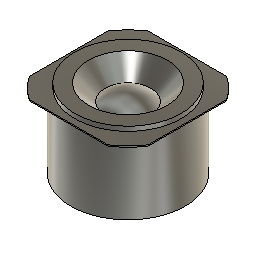
bc-4ndf34_phase_mount - thicker v5 v2 (Autodesk Fusion 360 archive; units mm, degrees)
design "bc-4ndf34-outline-parameterised"
Autodesk Fusion 360 part; units mm, degrees
sketch "Front frame" plane through (0, 0, 0) normal (0, 0, 1) x (1, 0, 0)
  line L0 (34.975, -53) -> (-34.975, -53)
  line L1 (-53, -34.975) -> (-53, 34.975)
  line L2 (-34.975, 53) -> (34.975, 53)
  line L3 (53, 34.975) -> (53, -34.975)
  line L4 (53, -53) -> (-53, 53) construction
  line L5 (-53, -53) -> (53, 53) construction
  arc A0 (53, 34.975) -> (34.975, 53) centre (0, 0) ccw
  arc A1 (53, 22.2991) -> (22.2991, 53) centre (0, 0) ccw
  arc A2 (34.975, -53) -> (53, -34.975) centre (0, 0) ccw
  arc A3 (22.2991, -53) -> (53, -22.2991) centre (0, 0) ccw
  arc A4 (-34.975, 53) -> (-53, 34.975) centre (0, 0) ccw
  arc A5 (-53, -34.975) -> (-34.975, -53) centre (0, 0) ccw
  arc A6 (-22.2991, 53) -> (-53, 22.2991) centre (0, 0) ccw
  arc A7 (-53, -22.2991) -> (-22.2991, -53) centre (0, 0) ccw
  circle A8 centre (0, 0) radius 51
  dimension "d1" = 127
  dimension "d2" = 115
  dimension "d3" = 106
  dimension "d4" = 106
  dimension "d15" = 102
  constraint coincident A0.centre A1.centre
  constraint horizontal L0
  constraint perpendicular L0 L1
  constraint parallel L0 L2
  constraint parallel L1 L3
  constraint coincident L4 A0.centre
  constraint coincident L5 A0.centre
  constraint coincident L2 A1.end
  constraint coincident L2 A6.start
  constraint coincident L3.start A4
  constraint concentric A0 A4
  constraint coincident L3 A3.end
  constraint coincident L3 A1.start
  constraint concentric A1 A6
  constraint coincident L0.start A4
  constraint concentric A2 A4
  constraint coincident L0 A7.end
  constraint coincident L0 A3.start
  constraint concentric A3 A6
  constraint coincident L1.start A4
  constraint concentric A4 A5
  constraint coincident L1 A6.end
  constraint coincident L1 A7.start
  constraint concentric A6 A7
  constraint concentric A4 A8
  measures "d1" diameter of A4
  measures "d2" diameter of A6
  measures "d3" distance of L4.end L5.end
  measures "d4" distance of L5.start L4.end
  measures "d15" diameter of A8
sketch "Side frame" plane through (0, 0, 0) normal (0, 1, 0) x (1, 0, 0)
  line L0 (-52.8388, 0) -> (53.1612, 0)
  line L1 (53.1612, 0) -> (53.1612, 1)
  line L2 (53.1612, 1) -> (-52.8388, 1)
  line L3 (-52.8388, 1) -> (-52.8388, 0)
  line L4 (51, 4) -> (-51, 4)
  line L5 (-51, 4) -> (-51, 1)
  line L6 (-51, 1) -> (51, 1)
  line L7 (51, 1) -> (51, 4)
  line L8 (51, 4) -> (-51, 1) construction
  line L9 (-51, 4) -> (51, 1) construction
  line L10 (51, 66) -> (-51, 66)
  line L11 (-51, 66) -> (-51, 0)
  line L12 (-51, 0) -> (51, 0)
  line L13 (51, 0) -> (51, 66)
  line L14 (51, 66) -> (-51, 0) construction
  line L15 (-51, 66) -> (51, 0) construction
  point P0 (0, 2.5)
  point P1 (0, 33)
  dimension "d5" = 106
  dimension "d6" = 1
  dimension "d8" = 2.5
  dimension "d9" = 102
  dimension "d10" = 3
  dimension "d13" = 102
  dimension "d14" = 66
  constraint horizontal L0
  constraint vertical L1
  constraint horizontal L2
  constraint vertical L3
  constraint horizontal L4
  constraint perpendicular L4 L5
  constraint parallel L4 L6
  constraint parallel L5 L7
  constraint coincident L8 P0
  constraint coincident L9 P0
  constraint horizontal L10
  constraint perpendicular L10 L11
  constraint parallel L10 L12
  constraint parallel L11 L13
  constraint coincident L14 P1
  constraint coincident L15 P1
  measures "d5" distance of L0.start L0.end
  measures "d6" distance of L0.start L2.end
  measures "d8" distance of origin P0
  measures "d9" distance of L5.end L6.end
  measures "d10" distance of L4.end L5.end
  measures "d13" distance of L11.end L12.end
  measures "d14" distance of L10.end L11.end
extrude "Extrude1" add sketch "Front frame" against normal blind 1 makes body 1
extrude "Extrude2" add sketch "Front frame" against normal blind 66 contours A8 bodies 1
sketch "cone surround" plane through (0, 0, 0) normal (0, 0, 1) x (1, 0, 0)
  circle A0 centre (0, 0) radius 47.5
  circle A1 centre (0, 0) radius 35
  circle A2 centre (0, 0) radius 20
  dimension "d20" = 95
  dimension "d21" = 70
  dimension "d22" = 40
  constraint coincident A0.centre A1.centre
  constraint concentric A0 A1
  measures "d20" diameter of A0
  measures "d21" diameter of A1
  measures "d22" diameter of A2
extrude "Extrude3" add sketch "cone surround" along normal blind 4 contours A0 bodies 1
sketch "cone sidewall" plane through (0, 0, 0) normal (0, 1, 0) x (1, 0, 0)
  circle A0 through (-20, 0, 0) (10, 0, 17.3205) (10, 0, -17.3205)
  circle A1 through (-35, 0, 0) (17.5, 0, 30.3109) (17.5, 0, -30.3109)
  line L0 (20, 0) -> (35, 0)
  line L1 (35, 10.1422) -> (35, -15)
  line L2 (35, -15) -> (9.8578, 10.1422)
  line L3 (40.0421, 10.1422) -> (0.0049, 10.1422)
  dimension "d35" = 15
  dimension "d43" = 45
  constraint horizontal L0
  constraint perpendicular L0 L1
  constraint horizontal L3
  constraint coincident L3 L2.end
  constraint coincident L0.start L2
  constraint coincident L3 L1.start
  constraint coincident L0.end L1
  measures "d35" distance of L0.end L1.end
  measures "d43" angle of L2 L3
move_face "OffsetFaces1" offset -65 1 faces at (10.7603, -1.7388, 0) on bodies 1
sketch "Sketch10" plane through (0, 0, 0) normal (0, 1, 0) x (1, 0, 0)
  line L0 (35.0027, 9.69) -> (0, 9.69)
  line L1 (0, 0) -> (0, 9.69)
  arc A0 (0, 0) -> (22.9486, 9.69) centre (-1.2492, 34.9777) ccw
  dimension "d38" = 70
  constraint coincident L1.start A0.start
  constraint perpendicular L0 L1
  constraint coincident L0 A0.end
  measures "d38" diameter of A0
revolve "Revolve2" add sketch "Sketch10" angle 360 about axis through (0, 0, 1.75) along (0, 0, 1) separate body makes body 2
move_body "Move4" bodies 2 to x (1, 0, 0) y (0, 1, 0) z (0, 0, 1) at (0, 0, -3)
revolve "Revolve3" add sketch "cone sidewall" angle 360 about axis through (0, 0, 1.75) along (0, 0, 1) separate body contours L0 L1 L2 makes body 3
move_face "MoveFace1" to x (1, 0, 0) y (0, 1, 0) z (0, 0, 1) at (0, 0, -15) 1 faces at (34.8261, -3.4849, 5) on bodies 3
move_body "Move5" bodies 3 to x (1, 0, 0) y (0, 1, 0) z (0, 0, 1) at (0, 0, -15)
move_body "Move6" bodies 3 to x (1, 0, 0) y (0, 1, 0) z (0, 0, 1) at (0, 0, 6)
move_face "MoveFace2" to x (1, 0, 0) y (0, 1, 0) z (0, 0, 1) at (0, 0, -2) 1 faces at (-11.5691, -29.4777, 2.6667) on bodies 3
extrude "Extrude4" add 1 faces at (-12.7748, -27.7902, -9) along direction (0, 0, -1) blind 2 draft 45 on bodies 3 bodies 3 1 2
equation "d22 = cone_inner_dia"
equation "dustcap_dia = 70 mm"
equation "d38 = dustcap_dia"
equation "cone_inner_dia = 40 mm"
named bodies: "speaker case - surround", "dustcap"
